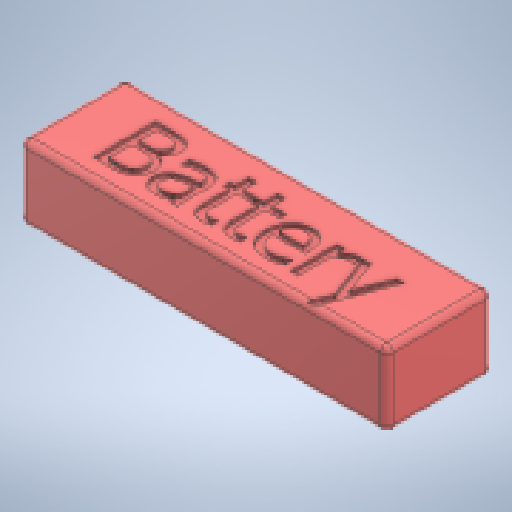
# Autodesk Inventor part: Battery Pack
Saved by Autodesk Inventor 2025.2 (Build 292293000, 293)
## iProperties
Created: 2022-10-23
Part Number: Battery Pack
Material: ABS Plastic
Document SubType Name: Modeling
Designer: chanh
Density: 1.06 g/cm^3
Appearance: Smooth - White
품번: 4
Author: chanh
Autodesk Inventor part; units mm, degrees
ref_plane "YZ Plane" through (0, 0, 0) normal (1, 0, 0) x (0, 1, 0)
ref_plane "XZ Plane" through (0, 0, 0) normal (0, 1, 0) x (-1, 0, 0)
ref_plane "XY Plane" through (0, 0, 0) normal (0, 0, 1) x (1, 0, 0)
sketch "Sketch1" plane through (0, 0, 0) normal (0, 1, 0) x (-1, 0, 0)
  line L0 (59, 17) -> (-59, 17)
  line L1 (-59, 17) -> (-59, -17)
  line L2 (-59, -17) -> (59, -17)
  line L3 (59, -17) -> (59, 17)
  line L4 (59, 17) -> (-59, -17) construction
  line L5 (-59, 17) -> (59, -17) construction
  point P0 (0, 0)
  dimension "d0" = 118
  dimension "d1" = 34
  constraints: 12 end point, 2 midpoint, 2 parallel, 1 horizontal, 1 perpendicular
  measures "d0" distance of L2.end L1.end
  measures "d1" distance of L1.end L0.end
extrude "Extrusion1" add sketch "Sketch1" along normal blind 24
sketch "Sketch2" plane through (0, 24, 0) normal (0, 1, 0) x (1, 0, 0)
  line L0 (-63.8755, 10.6972) -> (63.8755, 10.6972)
  line L1 (63.8755, 10.6972) -> (63.8755, -10.6972)
  line L2 (63.8755, -10.6972) -> (-63.8755, -10.6972)
  line L3 (-63.8755, -10.6972) -> (-63.8755, 10.6972)
  line L4 (-63.8755, 10.6972) -> (63.8755, -10.6972) construction
  line L5 (63.8755, 10.6972) -> (-63.8755, -10.6972) construction
  spline S0 degree 2 poles (-27.9822, -4.5546) (-27.9822, -6.0457) (-29.1167, -8.3309) (-30.0567, -9.0765) knots 0 0 0 1 2 2 2
  spline S1 degree 2 poles (-30.0567, -9.0765) (-31.1912, -9.9517) (-33.7682, -10.6972) (-35.8104, -10.6972) knots 0 0 0 1 2 2 2
  line L6 (-35.8104, -10.6972) -> (-41.5478, -10.6972)
  line L7 (-41.5478, -10.6972) -> (-41.5478, 9.3028)
  line L8 (-41.5478, 9.3028) -> (-36.248, 9.3028)
  spline S2 degree 2 poles (-36.248, 9.3028) (-34.1086, 9.3028) (-31.9692, 9.0273) (-30.9968, 8.4924) knots 0 0 0 1 2 2 2
  spline S3 degree 2 poles (-30.9968, 8.4924) (-29.9109, 7.9252) (-28.9222, 6.0613) (-28.9222, 4.7971) knots 0 0 0 1 2 2 2
  spline S4 degree 2 poles (-28.9222, 4.7971) (-28.9222, 3.3871) (-30.4133, 1.1504) (-31.7261, 0.5184) knots 0 0 0 1 2 2 2
  line L9 (-31.7261, 0.5184) -> (-31.7261, 0.4211)
  spline S5 degree 2 poles (-31.7261, 0.4211) (-29.9433, -0.0651) (-27.9822, -2.6421) (-27.9822, -4.5546) knots 0 0 0 1 2 2 2
  spline S6 degree 2 poles (-30.7536, -4.668) (-30.7536, -3.5335) (-31.4019, -2.0748) (-32.3744, -1.5562) knots 0 0 0 1 2 2 2
  spline S7 degree 2 poles (-32.3744, -1.5562) (-33.0065, -1.2321) (-34.4976, -1.0376) (-35.8752, -1.0376) knots 0 0 0 1 2 2 2
  line L10 (-35.8752, -1.0376) -> (-38.8898, -1.0376)
  line L11 (-38.8898, -1.0376) -> (-38.8898, -8.4282)
  line L12 (-38.8898, -8.4282) -> (-36.7342, -8.4282)
  spline S8 degree 2 poles (-36.7342, -8.4282) (-34.9838, -8.4282) (-32.9741, -8.104) (-32.1961, -7.5854) knots 0 0 0 1 2 2 2
  spline S9 degree 2 poles (-32.1961, -7.5854) (-31.4506, -7.0505) (-30.7536, -5.7215) (-30.7536, -4.668) knots 0 0 0 1 2 2 2
  spline S10 degree 2 poles (-31.6937, 4.4244) (-31.6937, 5.1375) (-32.1799, 6.2072) (-32.7147, 6.5151) knots 0 0 0 1 2 2 2
  spline S11 degree 2 poles (-32.7147, 6.5151) (-33.363, 6.8717) (-34.9352, 7.0338) (-36.3452, 7.0338) knots 0 0 0 1 2 2 2
  line L13 (-36.3452, 7.0338) -> (-38.8898, 7.0338)
  line L14 (-38.8898, 7.0338) -> (-38.8898, 1.1829)
  line L15 (-38.8898, 1.1829) -> (-35.8752, 1.1829)
  spline S12 degree 2 poles (-35.8752, 1.1829) (-34.6272, 1.1829) (-33.4441, 1.4422) (-32.812, 1.8474) knots 0 0 0 1 2 2 2
  spline S13 degree 2 poles (-32.812, 1.8474) (-32.1961, 2.2363) (-31.6937, 3.4843) (-31.6937, 4.4244) knots 0 0 0 1 2 2 2
  spline S14 degree 2 poles (-17.1718, -9.1089) (-17.4797, -9.3358) (-18.517, -10.1462) (-19.0032, -10.3893) knots 0 0 0 1 2 2 2
  spline S15 degree 2 poles (-19.0032, -10.3893) (-19.6677, -10.7458) (-20.9157, -11.1186) (-22.0502, -11.1186) knots 0 0 0 1 2 2 2
  spline S16 degree 2 poles (-22.0502, -11.1186) (-22.9741, -11.1186) (-24.6434, -10.4217) (-25.2755, -9.7896) knots 0 0 0 1 2 2 2
  spline S17 degree 2 poles (-25.2755, -9.7896) (-25.8752, -9.1737) (-26.6045, -7.3585) (-26.6045, -6.3536) knots 0 0 0 1 2 2 2
  spline S18 degree 2 poles (-26.6045, -6.3536) (-26.6045, -4.7977) (-25.2917, -2.5935) (-23.8655, -1.9614) knots 0 0 0 1 2 2 2
  spline S19 degree 2 poles (-23.8655, -1.9614) (-22.6013, -1.3779) (-19.1653, -0.9403) (-17.1718, -0.8269) knots 0 0 0 1 2 2 2
  line L16 (-17.1718, -0.8269) -> (-17.1718, -0.3406)
  spline S20 degree 2 poles (-17.1718, -0.3406) (-17.1718, 0.5346) (-17.7066, 1.6205) (-18.1929, 1.9284) knots 0 0 0 1 2 2 2
  spline S21 degree 2 poles (-18.1929, 1.9284) (-18.6791, 2.2363) (-20.0729, 2.4308) (-20.8185, 2.4308) knots 0 0 0 1 2 2 2
  spline S22 degree 2 poles (-20.8185, 2.4308) (-21.6937, 2.4308) (-24.06, 1.9122) (-25.2431, 1.4098) knots 0 0 0 1 2 2 2
  line L17 (-25.2431, 1.4098) -> (-25.389, 1.4098)
  line L18 (-25.389, 1.4098) -> (-25.389, 3.9867)
  spline S23 degree 2 poles (-25.389, 3.9867) (-24.6921, 4.1812) (-22.0827, 4.6675) (-20.8023, 4.6675) knots 0 0 0 1 2 2 2
  spline S24 degree 2 poles (-20.8023, 4.6675) (-19.2464, 4.6675) (-17.1232, 4.1812) (-16.2804, 3.5491) knots 0 0 0 1 2 2 2
  spline S25 degree 2 poles (-16.2804, 3.5491) (-15.4538, 2.9333) (-14.6434, 0.9722) (-14.6434, -0.4379) knots 0 0 0 1 2 2 2
  line L19 (-14.6434, -0.4379) -> (-14.6434, -10.6972)
  line L20 (-14.6434, -10.6972) -> (-17.1718, -10.6972)
  line L21 (-17.1718, -10.6972) -> (-17.1718, -9.1089)
  line L22 (-17.1718, -7.0019) -> (-17.1718, -2.8366)
  spline S26 degree 2 poles (-17.1718, -2.8366) (-18.0794, -2.9176) (-20.8185, -3.1932) (-21.6775, -3.4525) knots 0 0 0 1 2 2 2
  spline S27 degree 2 poles (-21.6775, -3.4525) (-22.6823, -3.7604) (-23.9951, -5.0408) (-23.9951, -6.1753) knots 0 0 0 1 2 2 2
  spline S28 degree 2 poles (-23.9951, -6.1753) (-23.9951, -7.4719) (-22.5365, -8.7847) (-21.1426, -8.7847) knots 0 0 0 1 2 2 2
  spline S29 degree 2 poles (-21.1426, -8.7847) (-19.9595, -8.7847) (-18.0146, -7.7637) (-17.1718, -7.0019) knots 0 0 0 1 2 2 2
  spline S30 degree 2 poles (-6.5559, -10.9889) (-8.6143, -10.9889) (-10.9319, -8.6389) (-10.9319, -6.0943) knots 0 0 0 1 2 2 2
  line L23 (-10.9319, -6.0943) -> (-10.9319, 2.2201)
  line L24 (-10.9319, 2.2201) -> (-12.6337, 2.2201)
  line L25 (-12.6337, 2.2201) -> (-12.6337, 4.3109)
  line L26 (-12.6337, 4.3109) -> (-10.9319, 4.3109)
  line L27 (-10.9319, 4.3109) -> (-10.9319, 8.6221)
  line L28 (-10.9319, 8.6221) -> (-8.4036, 8.6221)
  line L29 (-8.4036, 8.6221) -> (-8.4036, 4.3109)
  line L30 (-8.4036, 4.3109) -> (-3.752, 4.3109)
  line L31 (-3.752, 4.3109) -> (-3.752, 2.2201)
  line L32 (-3.752, 2.2201) -> (-8.4036, 2.2201)
  line L33 (-8.4036, 2.2201) -> (-8.4036, -4.9274)
  spline S31 degree 2 poles (-8.4036, -4.9274) (-8.4036, -6.0619) (-8.3225, -7.3098) (-8.047, -7.8447) knots 0 0 0 1 2 2 2
  spline S32 degree 2 poles (-8.047, -7.8447) (-7.8201, -8.3147) (-6.799, -8.7847) (-5.9238, -8.7847) knots 0 0 0 1 2 2 2
  spline S33 degree 2 poles (-5.9238, -8.7847) (-5.3079, -8.7847) (-4.1572, -8.412) (-3.8979, -8.2985) knots 0 0 0 1 2 2 2
  line L34 (-3.8979, -8.2985) -> (-3.752, -8.2985)
  line L35 (-3.752, -8.2985) -> (-3.752, -10.5675)
  spline S34 degree 2 poles (-3.752, -10.5675) (-4.4652, -10.762) (-5.9238, -10.9889) (-6.5559, -10.9889) knots 0 0 0 1 2 2 2
  spline S35 degree 2 poles (2.6499, -10.9889) (0.5916, -10.9889) (-1.7261, -8.6389) (-1.7261, -6.0943) knots 0 0 0 1 2 2 2
  line L36 (-1.7261, -6.0943) -> (-1.7261, 2.2201)
  line L37 (-1.7261, 2.2201) -> (-3.4279, 2.2201)
  line L38 (-3.4279, 2.2201) -> (-3.4279, 4.3109)
  line L39 (-3.4279, 4.3109) -> (-1.7261, 4.3109)
  line L40 (-1.7261, 4.3109) -> (-1.7261, 8.6221)
  line L41 (-1.7261, 8.6221) -> (0.8023, 8.6221)
  line L42 (0.8023, 8.6221) -> (0.8023, 4.3109)
  line L43 (0.8023, 4.3109) -> (5.4538, 4.3109)
  line L44 (5.4538, 4.3109) -> (5.4538, 2.2201)
  line L45 (5.4538, 2.2201) -> (0.8023, 2.2201)
  line L46 (0.8023, 2.2201) -> (0.8023, -4.9274)
  spline S36 degree 2 poles (0.8023, -4.9274) (0.8023, -6.0619) (0.8833, -7.3098) (1.1588, -7.8447) knots 0 0 0 1 2 2 2
  spline S37 degree 2 poles (1.1588, -7.8447) (1.3857, -8.3147) (2.4068, -8.7847) (3.282, -8.7847) knots 0 0 0 1 2 2 2
  spline S38 degree 2 poles (3.282, -8.7847) (3.8979, -8.7847) (5.0486, -8.412) (5.3079, -8.2985) knots 0 0 0 1 2 2 2
  line L47 (5.3079, -8.2985) -> (5.4538, -8.2985)
  line L48 (5.4538, -8.2985) -> (5.4538, -10.5675)
  spline S39 degree 2 poles (5.4538, -10.5675) (4.7407, -10.762) (3.282, -10.9889) (2.6499, -10.9889) knots 0 0 0 1 2 2 2
  spline S40 degree 2 poles (13.8331, -11.0376) (10.235, -11.0376) (6.2804, -7.0019) (6.2804, -3.2742) knots 0 0 0 1 2 2 2
  spline S41 degree 2 poles (6.2804, -3.2742) (6.2804, 0.3887) (10.1216, 4.7323) (13.2172, 4.7323) knots 0 0 0 1 2 2 2
  spline S42 degree 2 poles (13.2172, 4.7323) (14.611, 4.7323) (16.7666, 3.9219) (17.5608, 3.0629) knots 0 0 0 1 2 2 2
  spline S43 degree 2 poles (17.5608, 3.0629) (18.3712, 2.2039) (19.2301, -0.2758) (19.2301, -2.0748) knots 0 0 0 1 2 2 2
  line L49 (19.2301, -2.0748) -> (19.2301, -3.4525)
  line L50 (19.2301, -3.4525) -> (8.8412, -3.4525)
  spline S44 degree 2 poles (8.8412, -3.4525) (8.8412, -6.0619) (11.4668, -8.8333) (13.8006, -8.8333) knots 0 0 0 1 2 2 2
  spline S45 degree 2 poles (13.8006, -8.8333) (14.6272, -8.8333) (16.2318, -8.4606) (16.8801, -8.1688) knots 0 0 0 1 2 2 2
  spline S46 degree 2 poles (16.8801, -8.1688) (17.5608, -7.8447) (18.5008, -7.2774) (18.8088, -7.0181) knots 0 0 0 1 2 2 2
  line L51 (18.8088, -7.0181) -> (18.9546, -7.0181)
  line L52 (18.9546, -7.0181) -> (18.9546, -9.7734)
  spline S47 degree 2 poles (18.9546, -9.7734) (18.517, -9.9517) (17.188, -10.4703) (16.6694, -10.6162) knots 0 0 0 1 2 2 2
  spline S48 degree 2 poles (16.6694, -10.6162) (15.94, -10.8269) (14.7407, -11.0376) (13.8331, -11.0376) knots 0 0 0 1 2 2 2
  spline S49 degree 2 poles (16.7666, -1.5238) (16.7342, -0.5027) (16.3128, 0.9884) (15.9076, 1.4908) knots 0 0 0 1 2 2 2
  spline S50 degree 2 poles (15.9076, 1.4908) (15.47, 2.0581) (14.0924, 2.6577) (13.0713, 2.6577) knots 0 0 0 1 2 2 2
  spline S51 degree 2 poles (13.0713, 2.6577) (12.0665, 2.6577) (10.6564, 2.0581) (10.0729, 1.4746) knots 0 0 0 1 2 2 2
  spline S52 degree 2 poles (10.0729, 1.4746) (9.5057, 0.8749) (8.9222, -0.5675) (8.8412, -1.5238) knots 0 0 0 1 2 2 2
  line L53 (8.8412, -1.5238) -> (16.7666, -1.5238)
  line L54 (29.7488, 1.6043) -> (29.6191, 1.6043)
  spline S53 degree 2 poles (29.6191, 1.6043) (29.3274, 1.6853) (28.6953, 1.7177) (28.2577, 1.7177) knots 0 0 0 1 2 2 2
  spline S54 degree 2 poles (28.2577, 1.7177) (27.2366, 1.7177) (25.2269, 0.8263) (24.3193, -0.0489) knots 0 0 0 1 2 2 2
  line L55 (24.3193, -0.0489) -> (24.3193, -10.6972)
  line L56 (24.3193, -10.6972) -> (21.7909, -10.6972)
  line L57 (21.7909, -10.6972) -> (21.7909, 4.3109)
  line L58 (21.7909, 4.3109) -> (24.3193, 4.3109)
  line L59 (24.3193, 4.3109) -> (24.3193, 2.0743)
  spline S55 degree 2 poles (24.3193, 2.0743) (25.6969, 3.306) (27.7553, 4.3109) (28.7277, 4.3109) knots 0 0 0 1 2 2 2
  spline S56 degree 2 poles (28.7277, 4.3109) (29.1167, 4.3109) (29.5057, 4.2785) (29.7488, 4.2299) knots 0 0 0 1 2 2 2
  line L60 (29.7488, 4.2299) -> (29.7488, 1.6043)
  line L61 (43.4927, 4.3109) -> (35.4214, -16.2239)
  line L62 (35.4214, -16.2239) -> (32.7147, -16.2239)
  line L63 (32.7147, -16.2239) -> (35.4052, -9.9679)
  line L64 (35.4052, -9.9679) -> (29.9595, 4.3109)
  line L65 (29.9595, 4.3109) -> (32.6823, 4.3109)
  line L66 (32.6823, 4.3109) -> (36.7828, -6.8074)
  line L67 (36.7828, -6.8074) -> (40.8671, 4.3109)
  line L68 (40.8671, 4.3109) -> (43.4927, 4.3109)
  point P0 (0, 0)
  constraints: 12 end point, 2 horizontal, 2 midpoint, 2 parallel, 1 perpendicular
extrude "Extrusion2" cut sketch "Sketch2" against normal blind 1 contours L7 L8 S2 S3 S4 L9 S5 S0 S1 L2 | L61 L62 L63 L2 | L2 L63 L64 L65 L66 L67 L68 L61 | S16 S17 S18 S19 L16 S20 S21 S22 L17 L18 S23 S24 S25 L19 L2 L21 S14 S15 | L2 S15 S16 | L2 L57 L58 L59 S55 S56 L60 L54 S53 S54 L55 | S48 S40 L2 | L2 S40 S41 S42 S43 L49 L50 S44 S45 S46 L51 L52 S47 S48 | S30 L23 L24 L25 L26 L27 L28 L29 L30 L31 L32 L33 S31 S32 S33 L34 L35 S34 L2 | L2 S34 S30 | S39 S35 L2 | L2 S35 L36 L37 L38 L39 L40 L41 L42 L43 L44 L45 L46 S36 S37 S38 L47 L48 S39
fillet "Fillet1" radius 2 12 edges at (59, 24, 0) (0, 24, -17) (-59, 24, 0) (0, 24, 17) (0, 0, 17) (59, 12, 17) (-59, 12, 17) (-59, 0, 0) (-59, 12, -17) (0, 0, -17) (59, 12, -17) (59, 0, 0)
body "Solid1"
